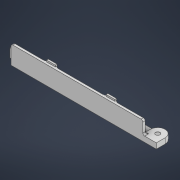
# Autodesk Inventor part: thinkpadcover
Saved by Autodesk Inventor 2022 (Build 260153000, 153)
## iProperties
Created: 2022-02-13
Part Number: thinkpadcover
Material: 一般
Document SubType Name: Modeling
Designer: shiokaze
Density: 1 g/cm^3
Appearance: 既定
Author: shiokaze
Autodesk Inventor part; units mm, degrees
ref_plane "YZ Plane" through (0, 0, 0) normal (1, 0, 0) x (0, 1, 0)
ref_plane "XZ Plane" through (0, 0, 0) normal (0, 1, 0) x (-1, 0, 0)
ref_plane "XY Plane" through (0, 0, 0) normal (0, 0, 1) x (1, 0, 0)
sketch "スケッチ1" plane through (0, 0, 0) normal (0, 1, 0) x (-1, 0, 0)
  line L0 (41.5, -4) -> (-41.5, -4)
  line L1 (-41.5, -4) -> (-41.5, 4)
  line L2 (-41.5, 4) -> (41.5, 4)
  line L3 (41.5, 4) -> (41.5, -4)
  circle A0 centre (-37.3, -1) radius 4.2
  line L4 (41.5, -4) -> (-41.5, 4) construction
  line L5 (-41.5, -4) -> (41.5, 4) construction
  point P0 (0, 0)
  point P1 (0, 0)
  point P2 (0, 0)
  point P3 (-41.5, -1)
  point P4 (-34.3606, -4)
  dimension "d0" = 83
  dimension "d1" = 8
  dimension "d2" = 8.4
  dimension "d3" = 5
  constraints: 12 end point, 2 midpoint, 2 parallel, 1 centre point, 1 coincident, 1 horizontal, 1 perpendicular, 1 tangent
  measures "d0" distance of L1.end L2.end
  measures "d1" distance of L0.end L1.end
  measures "d2" diameter of A0
  measures "d3" distance from line of A0.centre L2
extrude "押し出し1" add sketch "スケッチ1" along normal blind 0.9 contours L0 A0 L1 L2 L3 | A0 L0 | L0 A0
sketch "スケッチ2" plane through (0, 0.9, 0) normal (0, 1, 0) x (1, 0, 0)
  arc A0 (41.5, 1) -> (34.3606, 4) centre (37.3, 1) ccw projected
  line L0 (41.5, -4) -> (41.5, 1) projected
  circle A1 centre (37.3, 1) radius 4.2
  line L1 (33.1, 1) -> (33.1, -4)
  line L2 (-41.5, -4) -> (41.5, -4) projected
  line L3 (33.1, -4) -> (41.5, -4)
  point P0 (0, 0)
  constraints: 4 end point, 2 point on circle, 1 centre point, 1 coincident, 1 perpendicular, 1 tangent, 1 vertical
extrude "押し出し2" add sketch "スケッチ2" along normal blind 3.1 from surface at -0.9
sketch "スケッチ3" plane through (-41.5, 0, 4) normal (0, 0, 1) x (1, 0, 0)
  line L0 (0, 0) -> (0, 0.9) projected
  line L1 (0, 0) -> (75.3, 0)
  line L2 (75.3, 0) -> (75.3, 10.5)
  line L3 (75.3, 10.5) -> (0, 10.5)
  line L4 (0, 10.5) -> (0, 0)
  point P0 (41.5, 0)
  dimension "d8" = 75.3
  dimension "d9" = 10.5
  constraints: 8 end point, 2 parallel, 1 horizontal, 1 perpendicular
  measures "d8" distance of L3.end L2.end
  measures "d9" distance of L3.end L0.start
extrude "押し出し3" add sketch "スケッチ3" against normal blind 1.3
sketch "スケッチ4" plane through (-41.5, 0, 2.7) normal (0, 0, -1) x (-1, 0, 0)
  line L0 (-58, 11.4) -> (-53, 11.4)
  line L1 (-53, 11.4) -> (-53, 9.4)
  line L2 (-53, 9.4) -> (-58, 9.4)
  line L3 (-58, 9.4) -> (-58, 11.4)
  line L4 (-24, 11.4) -> (-19, 11.4)
  line L5 (-19, 11.4) -> (-19, 9.4)
  line L6 (-19, 9.4) -> (-24, 9.4)
  line L7 (-24, 9.4) -> (-24, 11.4)
  line L8 (0, 0.9) -> (0, 10.5) projected
  line L9 (-75.8606, 0) -> (0, 0) projected
  point P0 (-41.5, 0)
  point P1 (0, 2.9)
  dimension "d13" = 2
  dimension "d14" = 5
  dimension "d15" = 5
  dimension "d16" = 39
  dimension "d17" = 24
  dimension "d18" = 11.4
  constraints: 16 end point, 4 parallel, 2 horizontal, 2 perpendicular, 1 collinear, 1 point on line
  measures "d13" distance of L2.end L0.start
  measures "d14" distance of L1.end L2.end
  measures "d15" distance of L5.end L6.end
  measures "d16" distance between parallel lines of L5 L3
  measures "d17" distance between parallel lines of L8 L7
  measures "d18" distance between parallel lines of L9 L4
extrude "押し出し4" add sketch "スケッチ4" along normal blind 1
fillet "フィレット2" radius 2 9 edges at (33.428, 0.9, -2.627) (33.1, 2, 2.7) (33.1, 0.9, 0.85) (16.5, 9.95, 2.7) (11.5, 9.95, 2.7) (-17.5, 9.95, 2.7) (-22.5, 9.95, 2.7) (-20, 9.4, 2.7) (14, 9.4, 2.7)
sketch "スケッチ7" plane through (37.3, 3.1, -1) normal (0, 1, 0) x (1, 0, 0)
  arc A0 (4.2, 0) -> (-2.9394, 3) centre (0, 0) ccw projected
  point P0 (-37.3, -1)
  constraints: 1 coincident
hole "穴1" at (37.3, 3.1, -1) direction (0, -1, 0) diameter 2.5 depth 0.1 tip angle 118
fillet "フィレット3" radius 1 3 edges at (33.8, 10.5, 3.35) (-41.5, 10.5, 3.35) (-41.5, 0.45, -4)
fillet "フィレット4" radius 1 1 edges at (33.8, 3.1, 3.35)
fillet "フィレット5" radius 1 2 edges at (34.3, 3.1, 2.7) (32.45, 3.1, 2.7)
sketch "スケッチ8" plane through (-41.5, 0, 2.7) normal (0, 0, -1) x (-1, 0, 0)
  line L0 (-2, 7) -> (2, 7)
  line L1 (2, 7) -> (2, 2)
  line L2 (2, 2) -> (-2, 2)
  line L3 (-2, 2) -> (-2, 7)
  line L4 (-75.8606, 0) -> (-1, 0) projected
  line L5 (0, 0.9) -> (0, 9.5) projected
  line L6 (0, 0) -> (-83, 0) projected
  line L7 (-2, 2) -> (0, 2)
  line L8 (0, 2) -> (0, 0)
  line L9 (0, 0) -> (-2, 0)
  line L10 (-2, 0) -> (-2, 2)
  point P0 (-41.5, 0)
  point P1 (0, 2.9)
  point P2 (-2, 0)
  point P3 (0, 2)
  dimension "d41" = 7
  dimension "d42" = 2
  dimension "d43" = 4
  dimension "d44" = 5
  constraints: 16 end point, 4 parallel, 2 horizontal, 2 perpendicular
  measures "d41" distance between parallel lines of L4 L0
  measures "d42" distance between parallel lines of L5 L3
  measures "d43" distance between parallel lines of L1 L3
  measures "d44" distance between parallel lines of L0 L2
extrude "押し出し7" add sketch "スケッチ8" along normal blind 2.1
fillet "フィレット6" radius 2 2 edges at (32.5142, 1.4858, 2.1142) (-4.2, 0.9, 2.7)
fillet "フィレット7" radius 2 4 edges at (-39.5, 1.4858, 2.1142) (-39.5, 0.9, 0.65) (-39.5, 4.95, 2.7) (-40.5, 7, 2.7)
